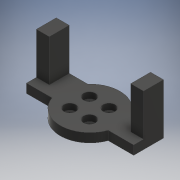
# Autodesk Inventor part: 腕-2
Saved by Autodesk Inventor 2017 (Build 210142000, 142)
## iProperties
Part Number: 腕-2
Material: 熱塑性塑膠樹脂
Document SubType Name: Modeling
Designer: Brian
Density: 1.28 g/cm^3
Appearance: 平滑 - 黑色
Mass: 9.13586 g
Surface Area: 48.4696 cm^2
Volume: 7.13739 cm^3
Author: Brian
Autodesk Inventor part; units mm, degrees
ref_plane "YZ Plane" through (0, 0, 0) normal (1, 0, 0) x (0, 1, 0)
ref_plane "XZ Plane" through (0, 0, 0) normal (0, 1, 0) x (-1, 0, 0)
ref_plane "XY Plane" through (0, 0, 0) normal (0, 0, 1) x (1, 0, 0)
sketch "草圖1" plane through (0, 0, 0) normal (0, 0, 1) x (1, 0, 0)
  circle A0 centre (0, 0) radius 10
  dimension "d0" = 20
  constraints: 1 centre point, 1 coincident
  measures "d0" diameter of A0
extrude "擠出1" add sketch "草圖1" along normal blind 5
ref_plane "工作平面1" through (0, 0, 0.5) normal (0, 0, -1) x (-1, 0, 0)
sketch "草圖4" plane through (0, 0, 0.5) normal (0, 0, -1) x (-1, 0, 0)
  circle A0 centre (-0.2588, 0) radius 15
  point P0 (0, 0)
  dimension "d18" = 30
  constraints: 1 centre point
  measures "d18" diameter of A0
extrude "擠出3" add sketch "草圖4" against normal up to surface (4.5 mm away)
sketch "草圖2" plane through (0, 0, 5) normal (0, 0, 1) x (1, 0, 0)
  circle A0 centre (0, 0) radius 7
  line L0 (-4.9497, -4.9497) -> (4.9497, -4.9497)
  line L1 (4.9497, -4.9497) -> (4.9497, 4.9497)
  line L2 (4.9497, 4.9497) -> (-4.9497, 4.9497)
  line L3 (-4.9497, 4.9497) -> (-4.9497, -4.9497)
  line L4 (-4.9497, -4.9497) -> (4.9497, 4.9497) construction
  line L5 (4.9497, -4.9497) -> (-4.9497, 4.9497) construction
  dimension "d3" = 14
  constraints: 12 end point, 2 midpoint, 2 parallel, 2 perpendicular, 1 coincident, 1 horizontal, 3 other
hole "孔1" at (4.9497, 4.9497, 5) at (-4.9497, 4.9497, 5) at (-4.9497, -4.9497, 5) at (4.9497, -4.9497, 5) direction (0, 0, -1) diameter 3.2 depth 8 tip angle 118 counterbore diameter 6 counterbore depth 3
sketch "草圖5" plane through (0.2588, 0, 5) normal (0, 0, 1) x (1, 0, 0)
  line L0 (-27, 10) -> (-10, 10)
  line L1 (-10, 10) -> (-10, -5)
  line L2 (-10, -5) -> (-27, -5)
  line L3 (-27, -5) -> (-27, 10)
  line L4 (10, 10) -> (27, 10)
  line L5 (27, 10) -> (27, -5)
  line L6 (27, -5) -> (10, -5)
  line L7 (10, -5) -> (10, 10)
  circle A0 centre (0, 0) radius 15 projected
  point P0 (-0.2588, 0)
  dimension "d21" = 10
  dimension "d22" = 10
  dimension "d23" = 10
  dimension "d24" = 15
  dimension "d27" = 17
  dimension "d28" = 17
  constraints: 16 end point, 4 parallel, 2 horizontal, 2 perpendicular, 2 point on line
  measures "d21" distance from line of point (-0.259, 0) L0
  measures "d22" distance from line of A0.centre L1
  measures "d23" distance from line of L7 A0.centre
  measures "d24" distance of L4.end L5.end
  measures "d27" distance of L0.start L0.end
  measures "d28" distance of L4.start L4.end
extrude "擠出4" add sketch "草圖5" against normal up to surface (4.5 mm away) contours L0 A0 L2 L3 | L0 L1 L2 A0 | A0 L6 L7 L4 | L4 L5 L6 A0
sketch "草圖6" plane through (0, 0, 5) normal (0, 0, 1) x (1, 0, 0)
  line L0 (-26.7412, 10) -> (-10.9215, 10) projected
  line L1 (-26.7412, 10) -> (-20.2412, 10)
  line L2 (-20.2412, 10) -> (-20.2412, 0)
  line L3 (-20.2412, 0) -> (-26.7412, 0)
  line L4 (-26.7412, 0) -> (-26.7412, 10)
  line L5 (27.2588, 10) -> (27.2588, -5) projected
  line L6 (27.2588, 10) -> (20.7588, 10)
  line L7 (20.7588, 10) -> (20.7588, 0)
  line L8 (20.7588, 0) -> (27.2588, 0)
  line L9 (27.2588, 0) -> (27.2588, 10)
  point P0 (0, 0)
  dimension "d29" = 41
  dimension "d30" = 10
  dimension "d31" = 10
  constraints: 16 end point, 4 parallel, 2 horizontal, 2 perpendicular, 1 collinear
  measures "d29" distance between parallel lines of L2 L7
  measures "d30" distance of L1.end L2.end
  measures "d31" distance of L6.end L7.end
extrude "擠出5" add sketch "草圖6" along normal blind 21
sketch "草圖7" plane through (-26.7412, 10, 0.5) normal (0, 1, 0) x (1, 0, 0)
  line L0 (2.7, -10.5) -> (51.3, -10.5)
  line L1 (51.3, -10.5) -> (51.3, -20.5)
  line L2 (51.3, -20.5) -> (2.7, -20.5)
  line L3 (2.7, -20.5) -> (2.7, -10.5)
  line L4 (0, 0) -> (0, -25.5) projected
  line L5 (6.5, -25.5) -> (0, -25.5) projected
  point P0 (26.7412, 0.5)
  dimension "d34" = 48.6
  dimension "d35" = 2.7
  dimension "d36" = 5
  dimension "d37" = 10
  constraints: 8 end point, 2 parallel, 1 horizontal, 1 perpendicular
  measures "d34" distance of L0.start L0.end
  measures "d35" distance between parallel lines of L4 L3
  measures "d36" distance between parallel lines of L5 L2
  measures "d37" distance of L2.end L0.start
hole "孔2" at (-24.0412, 10, 21) at (-24.0412, 10, 11) at (24.5588, 10, 21) at (24.5588, 10, 11) direction (0, -1, 0) diameter 3.2 depth 8 tip angle 118
